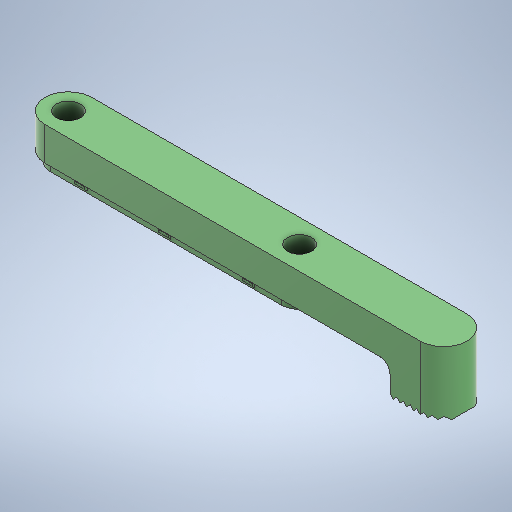
# Autodesk Inventor part: Gripper_attachment_1
Saved by Autodesk Inventor 2025.2 (Build 292293000, 293)
## iProperties
Created: 2025-04-18
Part Number: Gripper_attachment_1
Material: Generic
Document SubType Name: Modeling
Designer: caomi
Density: 1 g/cm^3
Appearance: Default
Author: caomi
Autodesk Inventor part; units mm, degrees
ref_plane "YZ Plane" through (0, 0, 0) normal (1, 0, 0) x (0, 1, 0)
ref_plane "XZ Plane" through (0, 0, 0) normal (0, 1, 0) x (-1, 0, 0)
ref_plane "XY Plane" through (0, 0, 0) normal (0, 0, 1) x (1, 0, 0)
sketch "Sketch1" plane through (0, 0, 0) normal (0, 1, 0) x (-1, 0, 0)
  line L0 (-41.5, -7) -> (41.5, -7)
  line L1 (41.5, -7) -> (41.5, 7)
  line L2 (41.5, 7) -> (-41.5, 7)
  line L3 (-41.5, 7) -> (-41.5, -7)
  line L4 (-41.5, -7) -> (41.5, 7) construction
  line L5 (41.5, -7) -> (-41.5, 7) construction
  circle A0 centre (34.5, 0) radius 3.6
  circle A1 centre (-34.5, 0) radius 3.6
  line L6 (0, 18.6517) -> (0, -10.4322) construction
  point P0 (0, 0)
  dimension "d0" = 14
  dimension "d1" = 83
  dimension "d2" = 7.2
  dimension "d3" = 69
  constraints: 14 end point, 2 centre point, 2 midpoint, 2 parallel, 1 equal radius, 1 horizontal, 1 horizontal alignment, 1 perpendicular, 1 point on line, 1 symmetric about line, 1 vertical
  measures "d0" distance of L0.end L1.end
  measures "d1" distance of L1.end L2.end
  measures "d2" diameter of A0
  measures "d3" distance of A1.centre A0.centre
extrude "Extrusion1" add sketch "Sketch1" along normal blind 10
fillet "Fillet1" radius 7 4 edges at (-41.5, 5, -7) (-41.5, 5, 7) (41.5, 5, -7) (41.5, 5, 7)
sketch "Sketch4" plane through (0, 0, 0) normal (0, -1, 0) x (1, 0, 0)
  arc A0 (34.5, -7) -> (34.5, 7) centre (34.5, 0) ccw projected
  line L0 (-34.5, 7) -> (34.5, 7) projected
  arc A1 (-34.5, 7) -> (-34.5, -7) centre (-34.5, 0) ccw projected
  line L1 (34.5, -7) -> (-34.5, -7) projected
  circle A2 centre (34.5, 0) radius 3.6 projected
  circle A3 centre (-34.5, 0) radius 3.6 projected
  arc A4 (34.5, -5.4) -> (34.5, 5.4) centre (34.5, 0) ccw
  line L2 (34.5, -5.4) -> (-34.5, -5.4)
  arc A5 (-34.5, 5.4) -> (-34.5, -5.4) centre (-34.5, 0) ccw
  line L3 (-34.5, 5.4) -> (34.5, 5.4)
  point P0 (0, 0)
  dimension "d8" = 1.6
  constraints: 4 end point, 4 point on circle, 2 centre point, 3 other
  measures "d8" distance between parallel lines of L0 L3
extrude "Extrusion2" add sketch "Sketch4" along normal blind 3 contours L2 A5 L3 A4
sketch "Sketch5" plane through (0, 0, 0) normal (1, 0, 0) x (0, 1, 0)
  line L0 (0, -5.4) -> (-3, -5.4) projected
  line L1 (-2.5, -5.4) -> (-1.5, -6.4)
  line L2 (-1.5, -6.4) -> (-0.5, -5.4)
  line L3 (-1.5, -6.4) -> (-1.5, -5.4) construction
  point P0 (0, 0)
  dimension "d11" = 1
  dimension "d12" = 45
  dimension "d13" = 0.5
  constraints: 6 end point, 2 point on line, 1 midpoint, 1 vertical, 1 other
  measures "d11" distance of L1.end L3.end
  measures "d12" angle of L0 L1
  measures "d13" distance of L0.end L1.start
extrude "Extrusion3" add sketch "Sketch5" along normal mid plane 3
fillet "Fillet2" radius 0.5 1 edges at (0, -1.5, -6.4)
pattern_linear "Rectangular Pattern1" count 3 spacing 25 along (-1, 0, 0) of "Extrusion3", "Fillet2" first direction both ways yes
mirror "Mirror1" about plane through (0, 0, 0) normal (0, 0, 1) of "Extrusion3", "Fillet2", "Rectangular Pattern1"
sketch "Sketch2" plane through (0, 10, 0) normal (0, 1, 0) x (1, 0, 0)
  line L0 (-34.5, -7) -> (34.5, -7) projected
  line L1 (34.5, -7) -> (84.5, -7)
  line L2 (84.5, -7) -> (84.5, 7)
  line L3 (34.5, 7) -> (-34.5, 7) projected
  line L4 (84.5, 7) -> (34.5, 7)
  circle A0 centre (34.5, 0) radius 3.6 projected
  arc A1 (34.5, -7) -> (34.5, 7) centre (34.5, 0) ccw projected
  point P0 (0, 0)
  dimension "d7" = 50
  constraints: 6 end point, 2 horizontal, 1 perpendicular
  measures "d7" distance from line of A0.centre L2
extrude "Extrusion4" add sketch "Sketch2" against normal up to surface (10 mm away) contours A1 L4 L2 L1
sketch "Sketch6" plane through (-34.5, 0, -7) normal (0, 0, -1) x (-1, 0, 0)
  line L0 (-119, 10) -> (-119, 0) projected
  line L1 (-119, 0) -> (-103, 0)
  line L2 (-103, 0) -> (-103, -8)
  line L3 (-103, -8) -> (-119, -8)
  line L4 (-119, -8) -> (-119, 0)
  line L5 (-119, -8) -> (-118, -9)
  line L6 (-118, -9) -> (-117, -8)
  line L7 (-118, -9) -> (-118, -8) construction
  line L8 (-116, -9) -> (-115, -8)
  line L9 (-117, -8) -> (-116, -9)
  line L10 (-114, -9) -> (-113, -8)
  line L11 (-115, -8) -> (-114, -9)
  line L12 (-112, -9) -> (-111, -8)
  line L13 (-113, -8) -> (-112, -9)
  line L14 (-110, -9) -> (-109, -8)
  line L15 (-111, -8) -> (-110, -9)
  line L16 (-108, -9) -> (-107, -8)
  line L17 (-109, -8) -> (-108, -9)
  line L18 (-106, -9) -> (-105, -8)
  line L19 (-107, -8) -> (-106, -9)
  line L20 (-104, -9) -> (-103, -8)
  line L21 (-105, -8) -> (-104, -9)
  point P0 (-34.5, 0)
  point P1 (-117, -8)
  point P2 (-115, -8)
  point P3 (-113, -8)
  point P4 (-111, -8)
  point P5 (-109, -8)
  point P6 (-107, -8)
  point P7 (-105, -8)
  point P8 (-103, -8)
  dimension "d22" = 16
  dimension "d23" = 1
  dimension "d24" = 45
  dimension "d27" = 2
  dimension "d32" = 8
  constraints: 42 end point, 2 horizontal, 2 parallel, 2 perpendicular, 2 point on line, 36 other
  measures "d22" distance of L2.end L3.end
  measures "d23" distance of L5.end L7.end
  measures "d24" angle of L3 L5
  measures "d27" distance of L5.end L8.start
  measures "d32" distance of L3.end L0.end
extrude "Extrusion5" add sketch "Sketch6" against normal up to surface (14 mm away)
fillet "Fillet3" radius 7 2 edges at (84.5, 1, -7) (84.5, 1, 7)
fillet "Fillet4" radius 3 1 edges at (68.5, 0, 0)
ref_plane "Work Plane1" through (0, 0, 0) normal (0, 0, 1) x (1, 0, 0)
equation "\"d6\" = 0.5 * d0"
equation "\"d35\" = 0.5 * d0"
body "Solid1"
